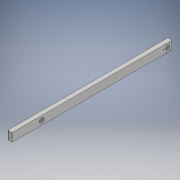
# Autodesk Inventor part: 41.75in Arm Beam Alternate (Left)
Saved by Autodesk Inventor 2018 (Build 220112000, 112)
## iProperties
Created: 2019-01-17
Part Number: 41.75in Arm Beam Alternate (Left)
Material: Generic
Document SubType Name: Modeling
Designer: Gabriel
Density: 1 g/cm^3
Appearance: Default
Author: Gabriel
Autodesk Inventor part; units mm, degrees
ref_plane "YZ Plane" through (0, 0, 0) normal (1, 0, 0) x (0, 1, 0)
ref_plane "XZ Plane" through (0, 0, 0) normal (0, 1, 0) x (-1, 0, 0)
ref_plane "XY Plane" through (0, 0, 0) normal (0, 0, 1) x (1, 0, 0)
sketch "Sketch1" plane through (0, 0, 0) normal (0, 0, 1) x (1, 0, 0)
  line L0 (-35.3228, 16.049) -> (-9.9228, 16.049)
  line L1 (-9.9228, 16.049) -> (-9.9228, -34.751)
  line L2 (-9.9228, -34.751) -> (-35.3228, -34.751)
  line L3 (-35.3228, -34.751) -> (-35.3228, 16.049)
  line L4 (-13.0978, 12.874) -> (-32.1478, 12.874)
  line L5 (-32.1478, 12.874) -> (-32.1478, -31.576)
  line L6 (-32.1478, -31.576) -> (-13.0978, -31.576)
  line L7 (-13.0978, -31.576) -> (-13.0978, 12.874)
  point P0 (0, 0)
  dimension "d0" = 25.4
  dimension "d1" = 50.8
  dimension "d2" = 3.175
  constraints: 16 end point, 4 parallel, 2 perpendicular, 1 horizontal, 3 other
  measures "d0" distance of L1.end L2.end
  measures "d1" distance of L0.end L1.end
  measures "d2" distance between parallel lines of L0 L4
extrude "Extrusion1" add sketch "Sketch1" along normal blind 965.2
sketch "Sketch2" plane through (-35.3228, -34.751, 0) normal (-1, 0, 0) x (0, 0, 1)
  line L0 (0, 0) -> (0, 50.8) construction
  line L1 (0, 25.4) -> (25.4, 25.4) construction
  circle A0 centre (25.4, 25.4) radius 14.2875
  point P0 (0, 34.751)
  dimension "d5" = 25.4
  dimension "d9" = 28.575
  constraints: 2 end point, 1 centre point, 1 coincident, 1 horizontal, 1 midpoint
  measures "d5" distance of L1.start L1.end
  measures "d9" diameter of A0
extrude "Extrusion2" cut sketch "Sketch2" against normal blind 12.7
sketch "Sketch3" plane through (-35.3228, -34.751, 0) normal (-1, 0, 0) x (0, 0, 1)
  line L0 (965.2, 50.8) -> (965.2, 0) construction
  line L1 (965.2, 25.4) -> (787.4, 25.4) construction
  circle A0 centre (787.4, 25.4) radius 14.2875
  point P0 (0, 34.751)
  dimension "d10" = 177.8
  dimension "d11" = 28.575
  constraints: 2 end point, 1 centre point, 1 coincident, 1 horizontal, 1 midpoint
  measures "d10" distance of L1.start L1.end
  measures "d11" diameter of A0
extrude "Extrusion3" cut sketch "Sketch3" against normal blind 25.4
sketch "Sketch6" plane through (-35.3228, -34.751, 0) normal (-1, 0, 0) x (0, 0, 1)
  line L0 (0, 47.625) -> (0, 3.175) construction
  line L1 (0, 25.4) -> (25.4, 25.4) construction
  line L2 (1.5875, 25.4) -> (13.4938, 46.0222)
  line L3 (13.4938, 46.0222) -> (37.3063, 46.0222)
  line L4 (37.3063, 46.0222) -> (49.2125, 25.4)
  line L5 (49.2125, 25.4) -> (37.3062, 4.7778)
  line L6 (37.3062, 4.7778) -> (13.4938, 4.7778)
  line L7 (13.4938, 4.7778) -> (1.5875, 25.4)
  circle A0 centre (13.4938, 46.0222) radius 2.5797
  circle A1 centre (37.3063, 46.0222) radius 2.5797
  circle A2 centre (49.2125, 25.4) radius 2.5797
  circle A3 centre (37.3062, 4.7778) radius 2.5797
  circle A4 centre (13.4938, 4.7778) radius 2.5797
  point P0 (0, 34.751)
  dimension "d25" = 25.4
  dimension "d26" = 47.625
  dimension "d27" = 5.1594
  dimension "d28" = 5.1594
  dimension "d29" = 5.1594
  dimension "d30" = 5.1594
  dimension "d31" = 5.1594
  constraints: 14 end point, 6 coincident, 5 centre point, 1 horizontal, 1 midpoint, 1 point on line, 13 other
  measures "d25" distance of L1.start L1.end
  measures "d26" distance of L4.end L2.start
  measures "d27" diameter of A0
  measures "d28" diameter of A1
  measures "d29" diameter of A2
  measures "d30" diameter of A3
  measures "d31" diameter of A4
extrude "Extrusion6" cut sketch "Sketch6" against normal blind 25.4 contours A0 L3 L2 | L2 L3 A0 | A4 L6 L7 | L7 L6 A4 | A1 L4 L3 | L3 L4 A1 | A3 L5 L6 | L6 L5 A3 | A2 L5 L4 | L4 L5 A2
sketch "Sketch7" plane through (-9.9228, -34.751, 0) normal (1, 0, 0) x (0, 0, -1)
  line L0 (0, 0) -> (0, 50.8) construction
  line L1 (0, 25.4) -> (-25.4, 25.4) construction
  circle A0 centre (-25.4, 25.4) radius 12.7
  point P0 (0, 34.751)
  dimension "d34" = 25.4
  dimension "d35" = 25.4
  constraints: 2 end point, 1 centre point, 1 coincident, 1 horizontal, 1 midpoint
  measures "d34" distance of L1.start L1.end
  measures "d35" diameter of A0
extrude "Extrusion7" cut sketch "Sketch7" against normal blind 12.7
body "Solid1"
